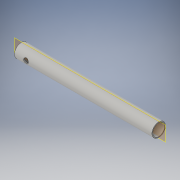
# Autodesk Inventor part: cArmPVC1_5inchSchedule120
Saved by Autodesk Inventor 2016 SP1 (Build 200210100, 210)
## iProperties
Created: 2016-01-12
Part Number: cArmPVC1_5inchSchedule120
Material: Generic
Document SubType Name: Modeling
Designer: steele
Density: 1 g/cm^3
Appearance: Default
Author: steele
Autodesk Inventor part; units mm, degrees
ref_plane "YZ Plane" through (0, 0, 0) normal (1, 0, 0) x (0, 1, 0)
ref_plane "XZ Plane" through (0, 0, 0) normal (0, 1, 0) x (-1, 0, 0)
sketch "Sketch3" plane through (0, 0, 0) normal (1, 0, 0) x (0, 1, 0)
  circle A0 centre (0, 0) radius 26.2509
  circle A1 centre (0, 0) radius 30.1625
  dimension "d10" = 60.325
  dimension "d11" = 52.5018
  constraints: 2 centre point, 2 coincident
  measures "d10" diameter of A1
  measures "d11" diameter of A0
extrude "Extrusion3" add sketch "Sketch3" along normal blind 609.6
ref_plane "Work Plane1" through (0, 0, 30.1625) normal (0, 0, 1) x (1, 0, 0)
sketch "Sketch5" plane through (0, 0, 30.1625) normal (0, 0, 1) x (1, 0, 0)
  circle A0 centre (50.8, 0) radius 10.668
  line L0 (0, 30.1625) -> (0, -30.1625) projected
  point P0 (0, 0)
  dimension "d25" = 21.336
  dimension "d26" = 50.8
  constraints: 1 centre point
  measures "d25" diameter of A0
  measures "d26" distance from line of A0.centre L0
extrude "Extrusion5" cut sketch "Sketch5" against normal through all
equation "\"d10\" = cArmOutsideDiam"
equation "\"d11\" = cArmInsideDiam"
equation "\"d12\" = cArmLength"
equation "\"d25\" = cArmAxelHoleDaim"
equation "\"d26\" = cArmSpacing"
equation "\"catapultArmWallThickness\" = 1.5875"
equation "\"catapultArmWidth\" = 50.8"
equation "\"catapultArmLength\" = 1219.2"
equation "\"cArmAxelHoleDaim\" = 21.336"
equation "\"catapultArmHoleDistanceFromEnd\" = 381"
equation "\"cArmInsideDiam\" = 52.5018"
equation "\"cArmOutsideDiam\" = 60.325"
equation "\"cArmLength\" = 609.6"
equation "\"cArmSpacing\" = 50.8"
body "Solid2"
